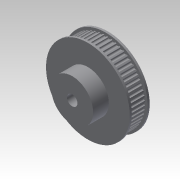
# Autodesk Inventor part: GT2 60T Drive Pulley
Saved by Autodesk Inventor 2020 (Build 240168000, 168)
## iProperties
Created: 2015-06-17
Part Number: GT2 60T Drive Pulley
Material: Generic
Document SubType Name: Modeling
Designer: Andrew
Density: 1 g/cm^3
Appearance: Default
Author: Andrew
Autodesk Inventor part; units mm, degrees
ref_plane "YZ Plane" through (0, 0, 0) normal (1, 0, 0) x (0, 1, 0)
ref_plane "XZ Plane" through (0, 0, 0) normal (0, 1, 0) x (-1, 0, 0)
ref_plane "XY Plane" through (0, 0, 0) normal (0, 0, 1) x (1, 0, 0)
sketch "Sketch1" plane through (0, 0, 0) normal (0, 0, 1) x (1, 0, 0)
  line L0 (0, 0) -> (0, 17) construction
  line L1 (0, 17) -> (2.5, 17) construction
  line L2 (2.5, 17) -> (20, 17)
  line L3 (20, 17) -> (20, 16)
  line L4 (20, 16) -> (18.85, 16)
  line L5 (18.85, 16) -> (18.85, 8.5)
  line L6 (18.85, 8.5) -> (20, 8.5)
  line L7 (2.5, 0) -> (2.5, 17)
  line L8 (2.5, 0) -> (10, 0)
  line L9 (10, 0) -> (10, 7.5)
  line L10 (10, 7.5) -> (20, 7.5)
  line L11 (20, 7.5) -> (20, 8.5)
  dimension "d0" = 2.5
  dimension "d1" = 7.5
  dimension "d4" = 1
  dimension "d6" = 18.85
  dimension "d15" = 20
  dimension "d16" = 7.5
  dimension "d17" = 10
  constraints: 24 end point, 8 perpendicular, 3 point on line, 1 collinear, 1 horizontal, 1 parallel, 1 vertical
  measures "d0" distance between parallel lines of L0 L7
  measures "d1" distance of L4.end L5.end
  measures "d4" distance between parallel lines of L2 L4
  measures "d6" distance between parallel lines of L0 L5
  measures "d15" distance between parallel lines of L0 L3
  measures "d16" distance of L8.end L9.end
  measures "d17" distance between parallel lines of L0 L9
revolve "Revolution1" add sketch "Sketch1" angle 360 about axis through (0, 0, 0) along (0, 1, 0)
sketch "Sketch2" plane through (0, 8.5, 0) normal (0, 1, 0) x (1, 0, 0)
  line L0 (0, 0) -> (0, -18.85)
  circle A0 centre (0, -18.85) radius 0.65
  dimension "d8" = 1.3
  dimension "d9" = 18.85
  constraints: 2 end point, 1 centre point, 1 coincident, 1 vertical
  measures "d8" diameter of A0
  measures "d9" distance of L0.start L0.end
extrude "Extrusion1" cut sketch "Sketch2" along normal up to surface (7.5 mm away)
pattern_circular "Circular Pattern1" count 60 over 360 about axis through (0, 12.25, 0) along (0, -1, 0) of "Extrusion1"
body "Solid1"
